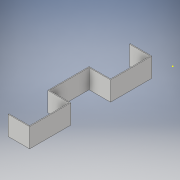
# Autodesk Inventor part: recreat2
Saved by Autodesk Inventor 2019 (Build 230136000, 136)
## iProperties
Created: 2021-11-03
Part Number: recreat2
Material: 一般
Document SubType Name: Modeling
Designer: yuta
Density: 1 g/cm^3
Appearance: 既定
Author: yuta
Autodesk Inventor part; units mm, degrees
ref_plane "YZ Plane" through (0, 0, 0) normal (1, 0, 0) x (0, 1, 0)
ref_plane "XZ Plane" through (0, 0, 0) normal (0, 1, 0) x (-1, 0, 0)
ref_plane "XY Plane" through (0, 0, 0) normal (0, 0, 1) x (1, 0, 0)
sketch "スケッチ1" plane through (0, 0, 0) normal (0, 1, 0) x (-1, 0, 0)
  line L0 (85.0374, 519.8276) -> (82.0374, 519.8276)
  line L1 (82.0374, 519.8276) -> (82.0374, 369.8276)
  line L2 (82.0374, 369.8276) -> (85.0374, 369.8276)
  line L3 (85.0374, 369.8276) -> (85.0374, 519.8276)
  line L4 (160.0374, 372.8276) -> (85.0374, 372.8276)
  line L5 (85.0374, 372.8276) -> (85.0374, 369.8276)
  line L6 (85.0374, 369.8276) -> (160.0374, 369.8276)
  line L7 (160.0374, 369.8276) -> (160.0374, 372.8276)
  line L8 (163.0374, 372.8276) -> (160.0374, 372.8276)
  line L9 (160.0374, 372.8276) -> (160.0374, 222.8276)
  line L10 (160.0374, 222.8276) -> (163.0374, 222.8276)
  line L11 (163.0374, 222.8276) -> (163.0374, 372.8276)
  line L12 (160.0374, 225.8276) -> (85.0374, 225.8276)
  line L13 (85.0374, 225.8276) -> (85.0374, 222.8276)
  line L14 (85.0374, 222.8276) -> (160.0374, 222.8276)
  line L15 (160.0374, 222.8276) -> (160.0374, 225.8276)
  line L16 (85.0374, 225.8276) -> (82.0374, 225.8276)
  line L17 (82.0374, 225.8276) -> (82.0374, 75.8276)
  line L18 (82.0374, 75.8276) -> (85.0374, 75.8276)
  line L19 (85.0374, 75.8276) -> (85.0374, 225.8276)
  point P0 (0, 0)
  dimension "d0" = 150
  dimension "d1" = 3
  dimension "d2" = 3
  dimension "d3" = 75
  dimension "d4" = 3
  dimension "d5" = 150
  dimension "d6" = 75
  dimension "d7" = 3
  dimension "d8" = 3
  dimension "d9" = 150
  constraints: 40 end point, 10 parallel, 8 collinear, 5 horizontal, 5 perpendicular
  measures "d0" distance of L2.end L0.start
  measures "d1" distance of L1.end L2.end
  measures "d2" distance of L4.end L5.end
  measures "d3" distance of L5.end L6.end
  measures "d4" distance of L10.end L9.end
  measures "d5" distance of L8.end L9.end
  measures "d6" distance of L14.end L13.end
  measures "d7" distance of L14.end L12.start
  measures "d8" distance of L18.end L17.end
  measures "d9" distance of L16.end L17.end
extrude "押し出し1" add sketch "スケッチ1" along normal blind 70
sketch "スケッチ2" plane through (-82.0374, 0, 519.8276) normal (1, 0, 0) x (0, 0, -1)
  point P0 (519.8276, 0)
sketch "スケッチ3" plane through (0, 70, 0) normal (0, 1, 0) x (1, 0, 0)
  line L0 (-160.0374, -516.8276) -> (-85.0374, -516.8276)
  line L1 (-85.0374, -516.8276) -> (-85.0374, -519.8276)
  line L2 (-85.0374, -519.8276) -> (-160.0374, -519.8276)
  line L3 (-160.0374, -519.8276) -> (-160.0374, -516.8276)
  line L4 (-85.0374, -372.8276) -> (-85.0374, -519.8276) projected
  line L5 (-85.0374, -519.8276) -> (-82.0374, -519.8276) projected
  line L6 (-160.0374, -75.8276) -> (-85.0374, -75.8276)
  line L7 (-85.0374, -75.8276) -> (-85.0374, -78.8276)
  line L8 (-85.0374, -78.8276) -> (-160.0374, -78.8276)
  line L9 (-160.0374, -78.8276) -> (-160.0374, -75.8276)
  line L10 (-85.0374, -75.8276) -> (-85.0374, -222.8276) projected
  line L11 (-82.0374, -75.8276) -> (-85.0374, -75.8276) projected
  point P0 (0, 0)
  dimension "d12" = 75
  dimension "d13" = 3
  dimension "d14" = 75
  dimension "d15" = 3
  constraints: 16 end point, 4 collinear, 4 parallel, 2 horizontal, 2 perpendicular
  measures "d12" distance of L1.end L2.end
  measures "d13" distance of L0.end L1.end
  measures "d14" distance of L7.end L8.end
  measures "d15" distance of L6.end L7.end
extrude "押し出し2" add sketch "スケッチ3" against normal blind 70
